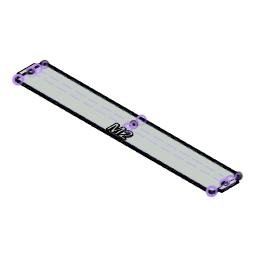
gridfinitybinlabel_parametric_blankPictogram v6 (Autodesk Fusion 360 design; units mm, degrees)
Autodesk Fusion 360 part; units mm, degrees
sketch "Sketch1" plane through (0, 0, 35.65) normal (0, 0, 1) x (-1, 0, 0)
  line L0 (-2.15, 2.65) -> (-39.9, 2.65)
  line L1 (-0.25, -3.35) -> (-0.25, -0.5)
  line L2 (-1.25, -0.5) -> (-1.25, 1.5)
  arc A0 (-1.25, 1.5) -> (-2.15, 2.4) centre (-2.15, 1.5) ccw
  line L3 (-2.15, 2.4) -> (-39.9, 2.4)
  line L4 (-1.25, -0.5) -> (-0.25, -0.5)
  line L5 (0, -3.35) -> (0, 0)
  line L6 (0, 0) -> (-1, 0)
  line L7 (-1, 0) -> (-1, 1.5)
  arc A1 (-1, 1.5) -> (-2.15, 2.65) centre (-2.15, 1.5) ccw
  line L8 (-39.9, -3.35) -> (-39.9, 2.65)
  line L9 (0, -3.35) -> (-39.9, -3.35)
  line L10 (0, 0) -> (-24, 0) construction
  line L11 (0, -3.35) -> (0, -6.7)
  line L12 (-1, -6.7) -> (-1, -8.2)
  line L13 (0, -3.35) -> (-39.9, -3.35)
  line L14 (-1.25, -6.2) -> (-0.25, -6.2)
  arc A2 (-2.15, -9.35) -> (-1, -8.2) centre (-2.15, -8.2) ccw
  line L15 (-2.15, -9.35) -> (-39.9, -9.35)
  line L16 (-1.25, -6.2) -> (-1.25, -8.2)
  line L17 (0, -6.7) -> (-1, -6.7)
  arc A3 (-2.15, -9.1) -> (-1.25, -8.2) centre (-2.15, -8.2) ccw
  line L18 (-0.25, -3.35) -> (-0.25, -6.2)
  line L19 (-2.15, -9.1) -> (-39.9, -9.1)
  line L20 (-39.9, -3.35) -> (-39.9, -9.35)
  line L21 (-78.55, -6.2) -> (-79.55, -6.2)
  line L22 (-79.8, -6.7) -> (-78.8, -6.7)
  line L23 (-77.65, -9.35) -> (-39.9, -9.35)
  line L24 (-79.8, -3.35) -> (-39.9, -3.35)
  line L25 (-78.8, 0) -> (-78.8, 1.5)
  line L26 (-77.65, 2.4) -> (-39.9, 2.4)
  line L27 (-78.55, -0.5) -> (-79.55, -0.5)
  line L28 (-77.65, 2.65) -> (-39.9, 2.65)
  arc A4 (-77.65, 2.4) -> (-78.55, 1.5) centre (-77.65, 1.5) ccw
  line L29 (-79.55, -3.35) -> (-79.55, -6.2)
  line L30 (-79.55, -3.35) -> (-79.55, -0.5)
  line L31 (-79.8, -3.35) -> (-39.9, -3.35)
  line L32 (-78.55, -6.2) -> (-78.55, -8.2)
  arc A5 (-78.55, -8.2) -> (-77.65, -9.1) centre (-77.65, -8.2) ccw
  line L33 (-79.8, -3.35) -> (-79.8, 0)
  line L34 (-39.9, -3.35) -> (-39.9, 2.65)
  line L35 (-79.8, 0) -> (-78.8, 0)
  arc A6 (-77.65, 2.65) -> (-78.8, 1.5) centre (-77.65, 1.5) ccw
  arc A7 (-78.8, -8.2) -> (-77.65, -9.35) centre (-77.65, -8.2) ccw
  line L36 (-78.55, -0.5) -> (-78.55, 1.5)
  line L37 (-77.65, -9.1) -> (-39.9, -9.1)
  line L38 (-78.8, -6.7) -> (-78.8, -8.2)
  line L39 (-39.9, -3.35) -> (-39.9, -9.35)
  line L40 (-79.8, -3.35) -> (-79.8, -6.7)
  point P0 (0, -6.7)
  point P1 (0, -6.7)
  point P2 (-79.8, -6.7)
  point P3 (-79.8, -6.7)
  point P4 (-79.8, 0)
  point P5 (-79.8, 0)
  dimension "d562" = 0.25
  dimension "d566" = 0.5
  dimension "d4" = 39.9
  dimension "d5" = 3.35
  dimension "d6" = 1
  dimension "d7" = 1
  dimension "d8" = 1.15
  dimension "d9" = 0.9
  dimension "d10" = 2
  dimension "d11" = 1.5
  dimension "d12" = 0.9
  dimension "d13" = 1.15
  constraint coincident L1 L4.end
  constraint perpendicular L1 L4
  constraint tangent L2 A0
  constraint tangent A0 L3
  constraint coincident A0.centre A1.centre
  constraint coincident L5.end L6.start
  constraint coincident L8 L3.end
  constraint coincident L9 L1.start
  constraint parallel L0 L3
  constraint perpendicular L6 L7
  constraint perpendicular L5 L9
  constraint parallel L9 L10
  constraint symmetric L5.end L9 P1
  constraint symmetric L0.start L9 A2.start
  constraint symmetric L2.end L9 L16.end
  constraint symmetric A0.end L9 A3.start
  constraint symmetric A0 L9 A3
  constraint symmetric L2.start L9 L14.start
  constraint symmetric L1.end L9 L14.end
  constraint symmetric L6.end L9 L12.start
  constraint symmetric L7.end L9 L12.end
  constraint symmetric A1 L9 A2
  constraint symmetric L5.start L9 L11.start
  constraint symmetric L8.start L9 L13.end
  constraint symmetric L0.end L9 L15.end
  constraint symmetric L3.end L9 L19.end
  constraint symmetric L9 L1.start L18.start
  constraint symmetric L9 L5.end P1
  constraint symmetric L5.end L20 P5
  constraint symmetric L0.start L20 L28.start
  constraint symmetric L2.end L20 A4.end
  constraint symmetric A0.end L20 L26.start
  constraint symmetric A0 L20 A4
  constraint symmetric L2.start L20 L27.start
  constraint symmetric L1.end L20 L27.end
  constraint symmetric L6.end L20 L25.start
  constraint symmetric L7.end L20 L25.end
  constraint symmetric A1 L20 A6
  constraint symmetric L5.start L20 L24.start
  constraint symmetric L8.start L20 L9.end
  constraint symmetric L0.end L20 L8.end
  constraint symmetric L3.end L20 L26.end
  constraint symmetric L1.start L20 L29.start
  constraint symmetric L15.end L20 L23.end
  constraint symmetric A3.start L20 A5.end
  constraint symmetric L12.end L20 A7.start
  constraint symmetric P1 L20 P3
  constraint symmetric L12.start L20 L22.end
  constraint symmetric L19.end L20 L37.end
  constraint symmetric L16.end L20 L32.end
  constraint symmetric L14.end L20 L21.end
  constraint symmetric A2.start L20 L23.start
  constraint symmetric L14.start L20 L21.start
  constraint symmetric A2 L20 A7
  constraint symmetric A3 L20 A5
  constraint perpendicular L3 L34
  measures "d562" distance of L1 L5
  measures "d566" distance of L4 L6
  measures "d4" distance of L5.start L8.start
  measures "d5" distance of L5.end L5.start
  measures "d6" distance of L5.end L6.end
  measures "d7" distance of L2.start L1.end
  measures "d8" radius of A1
  measures "d9" radius of A0
  measures "d10" distance of L2.end L2.start
  measures "d11" distance of L6.end L7.end
  measures "d12" distance of L2 A0.end
  measures "d13" horizontal distance of L0.start L7.end
extrude "Extrude1" add sketch "Sketch1" along normal blind 0.4
sketch "Sketch2" plane through (0, 0, 36.05) normal (0, 0, 1) x (-1, 0, 0)
  line L0 (-2.15, -8.6) -> (-77.65, -8.6)
  line L1 (-78.05, -8.2) -> (-78.05, 1.5)
  line L2 (-77.65, 1.9) -> (-2.15, 1.9)
  line L3 (-1.75, 1.5) -> (-1.75, -8.2)
  arc A0 (-2.15, -8.6) -> (-1.75, -8.2) centre (-2.15, -8.2) ccw
  arc A1 (-1.75, 1.5) -> (-2.15, 1.9) centre (-2.15, 1.5) ccw
  arc A2 (-77.65, 1.9) -> (-78.05, 1.5) centre (-77.65, 1.5) ccw
  arc A3 (-78.05, -8.2) -> (-77.65, -8.6) centre (-77.65, -8.2) ccw
  circle A4 centre (-1.75, -3.35) radius 0.75
  circle A5 centre (-78.05, -3.35) radius 0.75
  circle A6 centre (-1.75, -3.35) radius 1.25
  circle A7 centre (-78.05, -3.35) radius 1.25
  arc A8 (-2.15, -9.35) -> (-1, -8.2) centre (-2.15, -8.2) ccw
  line L4 (-1, -8.2) -> (-1, -6.7)
  line L5 (-1, -6.7) -> (0, -6.7)
  line L6 (0, -6.7) -> (0, 0)
  line L7 (0, 0) -> (-1, 0)
  line L8 (-1, 0) -> (-1, 1.5)
  arc A9 (-1, 1.5) -> (-2.15, 2.65) centre (-2.15, 1.5) ccw
  arc A10 (-77.65, 2.65) -> (-78.8, 1.5) centre (-77.65, 1.5) ccw
  line L9 (-2.15, 2.65) -> (-77.65, 2.65)
  arc A11 (-77.65, 2.65) -> (-78.8, 1.5) centre (-77.65, 1.5) ccw
  line L10 (-78.8, 1.5) -> (-78.8, 0)
  line L11 (-78.8, 0) -> (-79.8, 0)
  line L12 (-79.8, 0) -> (-79.8, -6.7)
  line L13 (-79.8, -6.7) -> (-78.8, -6.7)
  line L14 (-78.8, -6.7) -> (-78.8, -8.2)
  arc A12 (-78.8, -8.2) -> (-77.65, -9.35) centre (-77.65, -8.2) ccw
  line L15 (-77.65, -9.35) -> (-2.15, -9.35)
  point P0 (-2.15, -8.2)
  dimension "d517" = 1.5
  dimension "d518" = 2.5
  constraint horizontal L0
  constraint vertical L1
  constraint horizontal L2
  constraint vertical L3
  constraint tangent L0 A0
  constraint tangent L3 A0
  constraint tangent L3 A1
  constraint tangent L2 A1
  constraint equal A0 A1
  constraint tangent L2 A2
  constraint tangent L1 A2
  constraint equal A0 A2
  constraint tangent L1 A3
  constraint tangent L0 A3
  constraint equal A0 A3
  constraint midpoint L3 A4.centre
  constraint midpoint L1 A5.centre
  constraint concentric A4 A6
  constraint concentric A5 A7
  constraint equal A4 A5
  constraint equal A6 A7
  constraint coincident P0 A0.centre
  constraint concentric A2 A10
  measures "d517" diameter of A4
  measures "d518" diameter of A6
extrude "Extrude2" add sketch "Sketch2" along normal blind 0.4 contours L3 A4 A6 | L3 A4 A6 | L1 A5 A7 | L1 A5 A7 | L3 A4 | L3 A4 | L1 A5 | L1 A5 | A8 L4 L5 L6 L7 L8 A9 A10 L9 A11 L10 L11 L12 L13 L14 A12 L15
fillet "Fillet2" radius 1 6 edges at (1.75, 4.6, 36.25) (1.75, 2.1, 36.25) (1.75, 4.6, 36.25) (1.75, 2.1, 36.25) (78.05, 2.1, 36.25) (78.05, 4.6, 36.25)
extrude "Extrude4" cut sketch "Sketch2" along normal through all and the other way through all contours L3 A4 | L3 A4 | L1 A5 | L1 A5
fillet "Fillet1" radius 0.2 2 faces at (79.4667, 3.35, 36.45) (39.9, 1.35, 35.65)
sketch "Sketch3" plane through (0, 0, 36.05) normal (0, 0, 1) x (-1, 0, 0)
  line L0 (-77.65, -8.6) -> (-2.15, -8.6)
  line L1 (-2.15, 1.9) -> (-77.65, 1.9)
  line L2 (-2.15, -8.6) -> (-77.65, -8.6) construction
  line L3 (-77.65, -8.6) -> (-77.65, 1.9) construction
  line L4 (-77.65, 1.9) -> (-2.15, 1.9) construction
  line L5 (-2.15, 1.9) -> (-2.15, -8.6) construction
  line L6 (-2.15, -3.35) -> (-77.65, -3.35) construction
  arc A0 (-77.4944, -4.4698) -> (-78.05, -5.3656) centre (-77.05, -5.3656) ccw
  line L7 (-78.05, -5.3656) -> (-78.05, -8.2)
  arc A1 (-78.05, -8.2) -> (-77.65, -8.6) centre (-77.65, -8.2) ccw
  arc A2 (-2.15, -8.6) -> (-1.75, -8.2) centre (-2.15, -8.2) ccw
  line L8 (-1.75, -8.2) -> (-1.75, -5.3656)
  arc A3 (-1.75, -5.3656) -> (-2.3056, -4.4698) centre (-2.75, -5.3656) ccw
  arc A4 (-2.3056, -2.2302) -> (-2.3056, -4.4698) centre (-1.75, -3.35) ccw
  arc A5 (-2.3056, -2.2302) -> (-1.75, -1.3344) centre (-2.75, -1.3344) ccw
  line L9 (-1.75, -1.3344) -> (-1.75, 1.5)
  arc A6 (-1.75, 1.5) -> (-2.15, 1.9) centre (-2.15, 1.5) ccw
  arc A7 (-77.65, 1.9) -> (-78.05, 1.5) centre (-77.65, 1.5) ccw
  line L10 (-78.05, 1.5) -> (-78.05, -1.3344)
  arc A8 (-78.05, -1.3344) -> (-77.4944, -2.2302) centre (-77.05, -1.3344) ccw
  arc A9 (-77.4944, -4.4698) -> (-77.4944, -2.2302) centre (-78.05, -3.35) ccw
  line L11 (-2.15, -5.6) -> (-77.65, -5.6) construction
  line L12 (-39.9, -8.6) -> (-39.9, -5.6) construction
  line L13 (-39.9, -5.6) -> (-39.9, -3.35) construction
  line L14 (-34.3, -5.6) -> (-13, -5.6)
  line L15 (-13, -5.6) -> (-10, -5.6)
  line L16 (-2.15, 1.5) -> (-77.65, 1.5) construction
  line L17 (-77.65, 1.5) -> (-77.65, -3.35) construction
  line L18 (-77.65, -3.35) -> (-2.15, -3.35) construction
  line L19 (-2.15, -3.35) -> (-2.15, 1.5) construction
  line L20 (-39.9, -2.6) -> (-39.9, -5.6) construction
  line L21 (-13, -5.6) -> (-10, -5.6)
  point P0 (-34.3, -6.85)
  point P1 (-10, -8.1)
  point P2 (-6, -5.6)
  point P3 (-10, -3.1)
  point P4 (-34.3, -4.35)
  dimension "d21" = 3
  dimension "d22" = 0.4
  dimension "d26" = 2.5
  dimension "d38" = 75.5
  dimension "d43" = 4
  dimension "d44" = 0.4
  dimension "d67" = 0.4
  constraint horizontal L2
  constraint vertical L3
  constraint horizontal L4
  constraint vertical L5
  constraint midpoint L5 L6.start
  constraint midpoint L3 L6.end
  constraint coincident L5 L11.start
  constraint coincident L3 L11.end
  constraint perpendicular L3 L11
  constraint midpoint L2 L12.start
  constraint midpoint L11 L12.end
  constraint horizontal L14
  constraint coincident L11 L14.start
  constraint horizontal L15
  constraint coincident L1.start L4
  constraint coincident L5
  constraint coincident L6.end
  constraint symmetric L11 L12.start L20.start
  constraint symmetric L11 L12.end L13.start
  constraint symmetric L11 L14.end L15.start
  constraint symmetric L11 P0 P4
  constraint symmetric L11 L15.end L21.end
  constraint symmetric L11 P1 P3
  measures "d21" distance of L0 L11
  measures "d22" distance of L8 L11.start
  measures "d26" distance of L15.end P1
  measures "d38" distance of L0.end L0.start
  measures "d44" distance of L4 L16
  measures "d67" distance of L3 L7
sketch "Main Construction Geometry" plane through (0, 0, 36.05) normal (0, 0, 1) x (-1, 0, 0)
  arc A0 (-77.4944, -4.4698) -> (-78.05, -5.3656) centre (-77.05, -5.3656) ccw construction
  line L0 (-78.05, -5.3656) -> (-78.05, -8.2) construction
  arc A1 (-78.05, -8.2) -> (-77.65, -8.6) centre (-77.65, -8.2) ccw construction
  line L1 (-77.65, -8.6) -> (-2.15, -8.6) construction
  arc A2 (-2.15, -8.6) -> (-1.75, -8.2) centre (-2.15, -8.2) ccw construction
  line L2 (-1.75, -8.2) -> (-1.75, -5.3656) construction
  arc A3 (-1.75, -5.3656) -> (-2.3056, -4.4698) centre (-2.75, -5.3656) ccw construction
  arc A4 (-2.3056, -2.2302) -> (-2.3056, -4.4698) centre (-1.75, -3.35) ccw construction
  arc A5 (-2.3056, -2.2302) -> (-1.75, -1.3344) centre (-2.75, -1.3344) ccw construction
  line L3 (-1.75, -1.3344) -> (-1.75, 1.5) construction
  arc A6 (-1.75, 1.5) -> (-2.15, 1.9) centre (-2.15, 1.5) ccw construction
  line L4 (-2.15, 1.9) -> (-77.65, 1.9) construction
  arc A7 (-77.65, 1.9) -> (-78.05, 1.5) centre (-77.65, 1.5) ccw construction
  line L5 (-78.05, 1.5) -> (-78.05, -1.3344) construction
  arc A8 (-78.05, -1.3344) -> (-77.4944, -2.2302) centre (-77.05, -1.3344) ccw construction
  arc A9 (-77.4944, -4.4698) -> (-77.4944, -2.2302) centre (-78.05, -3.35) ccw construction
  line L6 (-2.15, -5.6) -> (-77.65, -5.6) construction
  line L7 (-2.15, 1.9) -> (-2.15, -8.6) construction
  line L8 (-2.15, -8.6) -> (-77.65, -8.6) construction
  line L9 (-39.9, -8.6) -> (-39.9, -5.6) construction
  line L10 (-39.9, -5.6) -> (-39.9, -3.35) construction
  line L11 (-2.15, -3.35) -> (-77.65, -3.35) construction
  line L12 (-77.65, -8.6) -> (-77.65, 1.9) construction
  line L13 (-2.15, 1.5) -> (-77.65, 1.5) construction
sketch "Pictogram" plane through (0, 0, 36.05) normal (0, 0, 1) x (-1, 0, 0)
  arc A0 (-77.4944, -4.4698) -> (-78.05, -5.3656) centre (-77.05, -5.3656) ccw
  line L0 (-78.05, -5.3656) -> (-78.05, -8.2)
  arc A1 (-78.05, -8.2) -> (-77.65, -8.6) centre (-77.65, -8.2) ccw
  line L1 (-77.65, -8.6) -> (-2.15, -8.6)
  arc A2 (-2.15, -8.6) -> (-1.75, -8.2) centre (-2.15, -8.2) ccw
  line L2 (-1.75, -8.2) -> (-1.75, -5.3656)
  arc A3 (-1.75, -5.3656) -> (-2.3056, -4.4698) centre (-2.75, -5.3656) ccw
  arc A4 (-2.3056, -2.2302) -> (-2.3056, -4.4698) centre (-1.75, -3.35) ccw
  arc A5 (-2.3056, -2.2302) -> (-1.75, -1.3344) centre (-2.75, -1.3344) ccw
  line L3 (-1.75, -1.3344) -> (-1.75, 1.5)
  arc A6 (-1.75, 1.5) -> (-2.15, 1.9) centre (-2.15, 1.5) ccw
  line L4 (-2.15, 1.9) -> (-77.65, 1.9)
  arc A7 (-77.65, 1.9) -> (-78.05, 1.5) centre (-77.65, 1.5) ccw
  line L5 (-78.05, 1.5) -> (-78.05, -1.3344)
  arc A8 (-78.05, -1.3344) -> (-77.4944, -2.2302) centre (-77.05, -1.3344) ccw
  arc A9 (-77.4944, -4.4698) -> (-77.4944, -2.2302) centre (-78.05, -3.35) ccw
sketch "Text" plane through (0, 0, 36.05) normal (0, 0, 1) x (-1, 0, 0)
  arc A0 (-77.4944, -4.4698) -> (-78.05, -5.3656) centre (-77.05, -5.3656) ccw
  line L0 (-78.05, -5.3656) -> (-78.05, -8.2)
  arc A1 (-78.05, -8.2) -> (-77.65, -8.6) centre (-77.65, -8.2) ccw
  line L1 (-77.65, -8.6) -> (-2.15, -8.6)
  arc A2 (-2.15, -8.6) -> (-1.75, -8.2) centre (-2.15, -8.2) ccw
  line L2 (-1.75, -8.2) -> (-1.75, -5.3656)
  arc A3 (-1.75, -5.3656) -> (-2.3056, -4.4698) centre (-2.75, -5.3656) ccw
  arc A4 (-2.3056, -2.2302) -> (-2.3056, -4.4698) centre (-1.75, -3.35) ccw
  arc A5 (-2.3056, -2.2302) -> (-1.75, -1.3344) centre (-2.75, -1.3344) ccw
  line L3 (-1.75, -1.3344) -> (-1.75, 1.5)
  arc A6 (-1.75, 1.5) -> (-2.15, 1.9) centre (-2.15, 1.5) ccw
  line L4 (-2.15, 1.9) -> (-77.65, 1.9)
  arc A7 (-77.65, 1.9) -> (-78.05, 1.5) centre (-77.65, 1.5) ccw
  line L5 (-78.05, 1.5) -> (-78.05, -1.3344)
  arc A8 (-78.05, -1.3344) -> (-77.4944, -2.2302) centre (-77.05, -1.3344) ccw
  arc A9 (-77.4944, -4.4698) -> (-77.4944, -2.2302) centre (-78.05, -3.35) ccw
  line L6 (-2.15, 1.5) -> (-77.65, 1.5) construction
  line L7 (-77.65, 1.5) -> (-77.65, -2.2355) construction
  line L8 (-77.65, -2.2355) -> (-2.15, -2.2355) construction
  line L9 (-2.15, -2.2355) -> (-2.15, 1.5) construction
  point P0 (-2.15, 1.5)
  point P1 (-77.65, 1.5)
  dimension "text_height" = 4
  text T0 "M2" font "Arial" height 4 bold align centre middle in box 75.5 x 3.7355 at (-2.15, 1.5) x (-1, 0) y (0, -1) spacing 1 kerned
  constraint coincident P0
  constraint coincident P1
extrude "Extrude6" add sketch "Text" along normal up to surface (0.4 mm away) text T0
extrude "Extrude3" [suppressed]
sketch "Skizze4" plane through (0, 0, 36.45) normal (0, 0, 1) x (-1, 0, 0)
  line L0 (-12.988, -6.85) -> (-12.988, -5.6) construction
  line L1 (-12.988, -5.6) -> (-34.3, -5.6) construction
  spline S0 degree 5 poles (-23.398, -6.85) (-23.3526, -6.8257) (-23.2673, -6.7758) (-23.156, -6.6971) (-23.0412, -6.5844) (-22.9541, -6.4303) (-22.9227, -6.2632) (-22.9431, -6.0841) (-23.0069, -5.8949) (-23.099, -5.6991) (-23.201, -5.5009) (-23.2931, -5.3051) (-23.3569, -5.1159) (-23.3773, -4.9368) (-23.3459, -4.7697) (-23.2588, -4.6156) (-23.144, -4.5029) (-23.0327, -4.4242) (-22.9474, -4.3743) (-22.902, -4.35) knots 0 0 0 0 0 0 0.066667 0.133333 0.2 0.266667 0.333333 0.4 0.466667 0.533333 0.6 0.666667 0.733333 0.8 0.866667 0.933333 1 1 1 1 1 1
  spline S1 degree 5 poles (-24.398, -6.85) (-24.3526, -6.8257) (-24.2673, -6.7758) (-24.156, -6.6971) (-24.0412, -6.5844) (-23.9541, -6.4303) (-23.9227, -6.2632) (-23.9431, -6.0841) (-24.0069, -5.8949) (-24.099, -5.6991) (-24.201, -5.5009) (-24.2931, -5.3051) (-24.3569, -5.1159) (-24.3773, -4.9368) (-24.3459, -4.7697) (-24.2588, -4.6156) (-24.144, -4.5029) (-24.0327, -4.4242) (-23.9474, -4.3743) (-23.902, -4.35) knots 0 0 0 0 0 0 0.066667 0.133333 0.2 0.266667 0.333333 0.4 0.466667 0.533333 0.6 0.666667 0.733333 0.8 0.866667 0.933333 1 1 1 1 1 1
  line L2 (-23.65, -5.6) -> (-22.95, -6.1)
  line L3 (-23.65, -5.6) -> (-23.95, -6.1)
  line L4 (-24.35, -5.1) -> (-23.65, -5.6)
  line L5 (-23.35, -5.1) -> (-23.65, -5.6)
  line L6 (-12.988, -5.6) -> (-12.988, -4.35) construction
  line L7 (-23.398, -6.85) -> (-24.398, -6.85)
  line L8 (-22.902, -4.35) -> (-23.902, -4.35)
  spline S2 degree 3 poles (-14.6415, -0.0138) (-14.6392, -0.1132) (-14.6345, -0.3083) (-14.5979, -0.4999) (-14.58, -0.5938) knots -0.058414 -0.058414 -0.058414 -0.058414 -0.028644 0 0 0 0
  spline S3 degree 3 poles (-14.58, -0.5938) (-14.5573, -0.6814) (-14.5135, -0.8507) (-14.4265, -1.0023) (-14.3846, -1.0754) knots -0.052175 -0.052175 -0.052175 -0.052175 -0.025167 0 0 0 0
  spline S4 degree 3 poles (-14.3846, -1.0754) (-14.3368, -1.1406) (-14.2412, -1.2707) (-14.106, -1.359) (-14.0385, -1.4031) knots -0.048014 -0.048014 -0.048014 -0.048014 -0.023977 0 0 0 0
  spline S5 degree 3 poles (-14.0385, -1.4031) (-13.9612, -1.4385) (-13.7973, -1.5136) (-13.6169, -1.5208) (-13.5215, -1.5246) knots -0.053559 -0.053559 -0.053559 -0.053559 -0.028317 0 0 0 0
  spline S6 degree 3 poles (-13.5215, -1.5246) (-13.4814, -1.5238) (-13.403, -1.5222) (-13.3256, -1.5094) (-13.2877, -1.5031) knots -0.023511 -0.023511 -0.023511 -0.023511 -0.011499 0 0 0 0
  spline S7 degree 3 poles (-13.2877, -1.5031) (-13.2509, -1.4948) (-13.1771, -1.4781) (-13.1073, -1.4486) (-13.0723, -1.4338) knots -0.022663 -0.022663 -0.022663 -0.022663 -0.011385 0 0 0 0
  spline S8 degree 3 poles (-13.0723, -1.4338) (-13.037, -1.4165) (-12.9644, -1.381) (-12.8975, -1.3356) (-12.8631, -1.3123) knots -0.024223 -0.024223 -0.024223 -0.024223 -0.01244 0 0 0 0
  spline S9 degree 3 poles (-12.8631, -1.3123) (-12.8276, -1.2858) (-12.754, -1.2309) (-12.688, -1.167) (-12.6538, -1.1338) knots -0.027525 -0.027525 -0.027525 -0.027525 -0.014261 0 0 0 0
  line L9 (-12.6538, -1.1338) -> (-12.6538, -2.6508)
  spline S10 degree 3 poles (-12.6538, -2.6508) (-12.6531, -2.6608) (-12.6515, -2.6808) (-12.6408, -2.6977) (-12.6354, -2.7062) knots -0.005919 -0.005919 -0.005919 -0.005919 -0.002959 0 0 0 0
  spline S11 degree 3 poles (-12.6354, -2.7062) (-12.6274, -2.7143) (-12.6095, -2.7327) (-12.5856, -2.7423) (-12.5723, -2.7477) knots -0.007625 -0.007625 -0.007625 -0.007625 -0.004249 0 0 0 0
  spline S12 degree 3 poles (-12.5723, -2.7477) (-12.5551, -2.7531) (-12.5164, -2.7654) (-12.4762, -2.7708) (-12.4538, -2.7738) knots -0.012151 -0.012151 -0.012151 -0.012151 -0.006747 0 0 0 0
  spline S13 degree 3 poles (-12.4538, -2.7738) (-12.4259, -2.7765) (-12.3635, -2.7825) (-12.3008, -2.7829) (-12.2662, -2.7831) knots -0.0188 -0.0188 -0.0188 -0.0188 -0.010387 0 0 0 0
  spline S14 degree 3 poles (-12.2662, -2.7831) (-12.2315, -2.7829) (-12.1688, -2.7825) (-12.1064, -2.7765) (-12.0785, -2.7738) knots -0.0188 -0.0188 -0.0188 -0.0188 -0.008413 0 0 0 0
  spline S15 degree 3 poles (-12.0785, -2.7738) (-12.0561, -2.7708) (-12.0159, -2.7654) (-11.9772, -2.7531) (-11.96, -2.7477) knots -0.012151 -0.012151 -0.012151 -0.012151 -0.005405 0 0 0 0
  spline S16 degree 3 poles (-11.96, -2.7477) (-11.9467, -2.7423) (-11.9228, -2.7327) (-11.9049, -2.7143) (-11.8969, -2.7062) knots -0.007625 -0.007625 -0.007625 -0.007625 -0.003376 0 0 0 0
  spline S17 degree 3 poles (-11.8969, -2.7062) (-11.8915, -2.6977) (-11.8808, -2.6808) (-11.8792, -2.6608) (-11.8785, -2.6508) knots -0.005919 -0.005919 -0.005919 -0.005919 -0.002959 0 0 0 0
  line L10 (-11.8785, -2.6508) -> (-11.8785, 1.3954)
  spline S18 degree 3 poles (-11.8785, 1.3954) (-11.879, 1.406) (-11.8799, 1.4261) (-11.8894, 1.4439) (-11.8938, 1.4523) knots -0.005963 -0.005963 -0.005963 -0.005963 -0.002824 0 0 0 0
  spline S19 degree 3 poles (-11.8938, 1.4523) (-11.9005, 1.4599) (-11.9154, 1.4769) (-11.9362, 1.4858) (-11.9477, 1.4908) knots -0.006691 -0.006691 -0.006691 -0.006691 -0.003699 0 0 0 0
  spline S20 degree 3 poles (-11.9477, 1.4908) (-11.9625, 1.4956) (-11.9955, 1.5064) (-12.0301, 1.5102) (-12.0492, 1.5123) knots -0.010404 -0.010404 -0.010404 -0.010404 -0.005755 0 0 0 0
  spline S21 degree 3 poles (-12.0492, 1.5123) (-12.0729, 1.5141) (-12.1257, 1.5181) (-12.1786, 1.5183) (-12.2077, 1.5185) knots -0.015862 -0.015862 -0.015862 -0.015862 -0.008732 0 0 0 0
  spline S22 degree 3 poles (-12.2077, 1.5185) (-12.2362, 1.5183) (-12.2885, 1.518) (-12.3408, 1.5141) (-12.3646, 1.5123) knots -0.015709 -0.015709 -0.015709 -0.015709 -0.007169 0 0 0 0
  spline S23 degree 3 poles (-12.3646, 1.5123) (-12.3841, 1.5102) (-12.4192, 1.5065) (-12.4528, 1.4956) (-12.4677, 1.4908) knots -0.010555 -0.010555 -0.010555 -0.010555 -0.004686 0 0 0 0
  spline S24 degree 3 poles (-12.4677, 1.4908) (-12.4793, 1.4858) (-12.5004, 1.4766) (-12.516, 1.4599) (-12.5231, 1.4523) knots -0.006807 -0.006807 -0.006807 -0.006807 -0.003074 0 0 0 0
  spline S25 degree 3 poles (-12.5231, 1.4523) (-12.528, 1.4439) (-12.5383, 1.4264) (-12.5394, 1.406) (-12.54, 1.3954) knots -0.006017 -0.006017 -0.006017 -0.006017 -0.003144 0 0 0 0
  line L11 (-12.54, 1.3954) -> (-12.54, 1.0969)
  spline S26 degree 3 poles (-12.54, 1.0969) (-12.5758, 1.1366) (-12.6441, 1.2125) (-12.7205, 1.2801) (-12.7569, 1.3123) knots -0.030591 -0.030591 -0.030591 -0.030591 -0.014564 0 0 0 0
  spline S27 degree 3 poles (-12.7569, 1.3123) (-12.7919, 1.3405) (-12.8599, 1.3953) (-12.9356, 1.4388) (-12.9723, 1.46) knots -0.026151 -0.026151 -0.026151 -0.026151 -0.012704 0 0 0 0
  spline S28 degree 3 poles (-12.9723, 1.46) (-13.0091, 1.4781) (-13.0826, 1.5143) (-13.1619, 1.5345) (-13.2015, 1.5446) knots -0.024494 -0.024494 -0.024494 -0.024494 -0.01222 0 0 0 0
  spline S29 degree 3 poles (-13.2015, 1.5446) (-13.243, 1.5522) (-13.3284, 1.568) (-13.4153, 1.5698) (-13.46, 1.5708) knots -0.026016 -0.026016 -0.026016 -0.026016 -0.013401 0 0 0 0
  spline S30 degree 3 poles (-13.46, 1.5708) (-13.5495, 1.5668) (-13.7228, 1.5591) (-13.8827, 1.4923) (-13.96, 1.46) knots -0.05157 -0.05157 -0.05157 -0.05157 -0.024925 0 0 0 0
  spline S31 degree 3 poles (-13.96, 1.46) (-14.0307, 1.4188) (-14.1734, 1.3356) (-14.278, 1.2076) (-14.3308, 1.1431) knots -0.049129 -0.049129 -0.049129 -0.049129 -0.024796 0 0 0 0
  spline S32 degree 3 poles (-14.3308, 1.1431) (-14.3786, 1.0688) (-14.4786, 0.9135) (-14.5331, 0.7368) (-14.5615, 0.6446) knots -0.055158 -0.055158 -0.055158 -0.055158 -0.028785 0 0 0 0
  spline S33 degree 3 poles (-14.5615, 0.6446) (-14.5849, 0.5414) (-14.6338, 0.3247) (-14.6389, 0.1026) (-14.6415, -0.0138) knots -0.066478 -0.066478 -0.066478 -0.066478 -0.034827 0 0 0 0
  spline S34 degree 3 poles (-13.8385, 0.0415) (-13.8372, 0.094) (-13.8345, 0.1993) (-13.8167, 0.3032) (-13.8077, 0.3554) knots -0.031572 -0.031572 -0.031572 -0.031572 -0.015861 0 0 0 0
  spline S35 degree 3 poles (-13.8077, 0.3554) (-13.7962, 0.4056) (-13.774, 0.5029) (-13.7293, 0.5922) (-13.7077, 0.6354) knots -0.029827 -0.029827 -0.029827 -0.029827 -0.014442 0 0 0 0
  spline S36 degree 3 poles (-13.7077, 0.6354) (-13.6835, 0.6742) (-13.6362, 0.7502) (-13.5675, 0.8074) (-13.5338, 0.8354) knots -0.026652 -0.026652 -0.026652 -0.026652 -0.013037 0 0 0 0
  spline S37 degree 3 poles (-13.5338, 0.8354) (-13.4961, 0.8578) (-13.4175, 0.9045) (-13.326, 0.9096) (-13.2785, 0.9123) knots -0.027024 -0.027024 -0.027024 -0.027024 -0.014055 0 0 0 0
  spline S38 degree 3 poles (-13.2785, 0.9123) (-13.2239, 0.9072) (-13.1109, 0.8965) (-13.0155, 0.8349) (-12.9662, 0.8031) knots -0.033522 -0.033522 -0.033522 -0.033522 -0.017328 0 0 0 0
  spline S39 degree 3 poles (-12.9662, 0.8031) (-12.9138, 0.7598) (-12.7986, 0.6647) (-12.7049, 0.5481) (-12.6538, 0.4846) knots -0.044706 -0.044706 -0.044706 -0.044706 -0.024376 0 0 0 0
  line L12 (-12.6538, 0.4846) -> (-12.6538, -0.4262)
  spline S40 degree 3 poles (-12.6538, -0.4262) (-12.6832, -0.4644) (-12.7381, -0.5362) (-12.8002, -0.6017) (-12.8292, -0.6323) knots -0.027083 -0.027083 -0.027083 -0.027083 -0.012631 0 0 0 0
  spline S41 degree 3 poles (-12.8292, -0.6323) (-12.8559, -0.6582) (-12.9065, -0.7072) (-12.9637, -0.7483) (-12.9908, -0.7677) knots -0.021102 -0.021102 -0.021102 -0.021102 -0.009969 0 0 0 0
  spline S42 degree 3 poles (-12.9908, -0.7677) (-13.016, -0.7836) (-13.0641, -0.814) (-13.1177, -0.8327) (-13.1431, -0.8415) knots -0.016975 -0.016975 -0.016975 -0.016975 -0.00805 0 0 0 0
  spline S43 degree 3 poles (-13.1431, -0.8415) (-13.1678, -0.8478) (-13.2173, -0.8604) (-13.2683, -0.8622) (-13.2938, -0.8631) knots -0.015269 -0.015269 -0.015269 -0.015269 -0.007634 0 0 0 0
  spline S44 degree 3 poles (-13.2938, -0.8631) (-13.3428, -0.8607) (-13.4357, -0.8562) (-13.5159, -0.8097) (-13.5538, -0.7877) knots -0.027422 -0.027422 -0.027422 -0.027422 -0.012953 0 0 0 0
  spline S45 degree 3 poles (-13.5538, -0.7877) (-13.5869, -0.7599) (-13.6548, -0.7028) (-13.6989, -0.6257) (-13.7215, -0.5862) knots -0.026401 -0.026401 -0.026401 -0.026401 -0.013559 0 0 0 0
  spline S46 degree 3 poles (-13.7215, -0.5862) (-13.7416, -0.5416) (-13.7834, -0.4488) (-13.8024, -0.3489) (-13.8123, -0.2969) knots -0.030408 -0.030408 -0.030408 -0.030408 -0.015795 0 0 0 0
  spline S47 degree 3 poles (-13.8123, -0.2969) (-13.8199, -0.2416) (-13.8354, -0.1293) (-13.8374, -0.016) (-13.8385, 0.0415) knots -0.033974 -0.033974 -0.033974 -0.033974 -0.017243 0 0 0 0
  line L13 (-19.1462, 1.4046) -> (-19.1462, -0.4415)
  spline S48 degree 3 poles (-19.1462, -0.4415) (-19.1442, -0.53) (-19.1405, -0.6958) (-19.0982, -0.856) (-19.0785, -0.9308) knots -0.049542 -0.049542 -0.049542 -0.049542 -0.023103 0 0 0 0
  spline S49 degree 3 poles (-19.0785, -0.9308) (-19.0532, -0.9958) (-19.0039, -1.1226) (-18.9092, -1.2201) (-18.8631, -1.2677) knots -0.040352 -0.040352 -0.040352 -0.040352 -0.01967 0 0 0 0
  spline S50 degree 3 poles (-18.8631, -1.2677) (-18.8088, -1.3089) (-18.6946, -1.3955) (-18.5578, -1.4388) (-18.4862, -1.4615) knots -0.042665 -0.042665 -0.042665 -0.042665 -0.022364 0 0 0 0
  spline S51 degree 3 poles (-18.4862, -1.4615) (-18.4022, -1.4799) (-18.2204, -1.5197) (-18.0341, -1.5229) (-17.9338, -1.5246) knots -0.055711 -0.055711 -0.055711 -0.055711 -0.030003 0 0 0 0
  spline S52 degree 3 poles (-17.9338, -1.5246) (-17.8741, -1.5235) (-17.7561, -1.5212) (-17.6393, -1.5039) (-17.5815, -1.4954) knots -0.035384 -0.035384 -0.035384 -0.035384 -0.017484 0 0 0 0
  spline S53 degree 3 poles (-17.5815, -1.4954) (-17.5266, -1.4852) (-17.4201, -1.4655) (-17.3163, -1.4348) (-17.2662, -1.42) knots -0.032447 -0.032447 -0.032447 -0.032447 -0.015686 0 0 0 0
  spline S54 degree 3 poles (-17.2662, -1.42) (-17.2207, -1.4049) (-17.1347, -1.3763) (-17.0525, -1.338) (-17.0138, -1.32) knots -0.02716 -0.02716 -0.02716 -0.02716 -0.012793 0 0 0 0
  spline S55 degree 3 poles (-17.0138, -1.32) (-16.9824, -1.3041) (-16.9284, -1.2769) (-16.8824, -1.2379) (-16.8631, -1.2215) knots -0.018062 -0.018062 -0.018062 -0.018062 -0.007557 0 0 0 0
  spline S56 degree 3 poles (-16.8631, -1.2215) (-16.8499, -1.2064) (-16.8241, -1.1767) (-16.811, -1.1397) (-16.8046, -1.1215) knots -0.011676 -0.011676 -0.011676 -0.011676 -0.005722 0 0 0 0
  spline S57 degree 3 poles (-16.8046, -1.1215) (-16.8001, -1.0998) (-16.7899, -1.0501) (-16.7895, -0.9993) (-16.7892, -0.9708) knots -0.015187 -0.015187 -0.015187 -0.015187 -0.008547 0 0 0 0
  spline S58 degree 3 poles (-16.7892, -0.9708) (-16.7895, -0.9482) (-16.7901, -0.9049) (-16.7958, -0.862) (-16.7985, -0.8415) knots -0.012966 -0.012966 -0.012966 -0.012966 -0.006193 0 0 0 0
  spline S59 degree 3 poles (-16.7985, -0.8415) (-16.8016, -0.8234) (-16.8074, -0.7898) (-16.8192, -0.7578) (-16.8246, -0.7431) knots -0.010206 -0.010206 -0.010206 -0.010206 -0.004707 0 0 0 0
  spline S60 degree 3 poles (-16.8246, -0.7431) (-16.8303, -0.7308) (-16.8411, -0.7077) (-16.8592, -0.6899) (-16.8677, -0.6815) knots -0.007567 -0.007567 -0.007567 -0.007567 -0.003539 0 0 0 0
  spline S61 degree 3 poles (-16.8677, -0.6815) (-16.8767, -0.6753) (-16.8948, -0.6627) (-16.9167, -0.6609) (-16.9277, -0.66) knots -0.006477 -0.006477 -0.006477 -0.006477 -0.003238 0 0 0 0
  spline S62 degree 3 poles (-16.9277, -0.66) (-16.9468, -0.6627) (-16.992, -0.669) (-17.0322, -0.6906) (-17.0554, -0.7031) knots -0.01357 -0.01357 -0.01357 -0.01357 -0.007814 0 0 0 0
  spline S63 degree 3 poles (-17.0554, -0.7031) (-17.0846, -0.7185) (-17.1488, -0.7523) (-17.2148, -0.7822) (-17.2508, -0.7985) knots -0.021747 -0.021747 -0.021747 -0.021747 -0.011839 0 0 0 0
  spline S64 degree 3 poles (-17.2508, -0.7985) (-17.2924, -0.8159) (-17.3804, -0.8526) (-17.4719, -0.8796) (-17.52, -0.8938) knots -0.028581 -0.028581 -0.028581 -0.028581 -0.015047 0 0 0 0
  spline S65 degree 3 poles (-17.52, -0.8938) (-17.574, -0.9064) (-17.6878, -0.9329) (-17.8047, -0.9355) (-17.8662, -0.9369) knots -0.034965 -0.034965 -0.034965 -0.034965 -0.018378 0 0 0 0
  spline S66 degree 3 poles (-17.8662, -0.9369) (-17.9116, -0.9361) (-17.9954, -0.9347) (-18.0767, -0.9151) (-18.1138, -0.9062) knots -0.025026 -0.025026 -0.025026 -0.025026 -0.011428 0 0 0 0
  spline S67 degree 3 poles (-18.1138, -0.9062) (-18.145, -0.895) (-18.2047, -0.8737) (-18.2515, -0.8311) (-18.2738, -0.8108) knots -0.018792 -0.018792 -0.018792 -0.018792 -0.008974 0 0 0 0
  spline S68 degree 3 poles (-18.2738, -0.8108) (-18.2926, -0.7874) (-18.3313, -0.7389) (-18.3502, -0.6798) (-18.36, -0.6492) knots -0.018446 -0.018446 -0.018446 -0.018446 -0.009535 0 0 0 0
  spline S69 degree 3 poles (-18.36, -0.6492) (-18.3676, -0.6144) (-18.3839, -0.5399) (-18.3854, -0.4636) (-18.3862, -0.4231) knots -0.022815 -0.022815 -0.022815 -0.022815 -0.012133 0 0 0 0
  line L14 (-18.3862, -0.4231) -> (-18.3862, -0.2569)
  line L15 (-18.3862, -0.2569) -> (-18.1185, -0.2569)
  spline S70 degree 3 poles (-18.1185, -0.2569) (-18.0036, -0.2553) (-17.7878, -0.2522) (-17.5749, -0.2177) (-17.4754, -0.2015) knots -0.064622 -0.064622 -0.064622 -0.064622 -0.03021 0 0 0 0
  spline S71 degree 3 poles (-17.4754, -0.2015) (-17.3892, -0.182) (-17.2272, -0.1452) (-17.0808, -0.0672) (-17.0123, -0.0308) knots -0.049551 -0.049551 -0.049551 -0.049551 -0.023172 0 0 0 0
  spline S72 degree 3 poles (-17.0123, -0.0308) (-16.9545, 0.0095) (-16.8415, 0.0883) (-16.7681, 0.2047) (-16.7323, 0.2615) knots -0.040845 -0.040845 -0.040845 -0.040845 -0.019941 0 0 0 0
  spline S73 degree 3 poles (-16.7323, 0.2615) (-16.705, 0.3249) (-16.6475, 0.4578) (-16.6416, 0.6026) (-16.6385, 0.6785) knots -0.04306 -0.04306 -0.04306 -0.04306 -0.022545 0 0 0 0
  spline S74 degree 3 poles (-16.6385, 0.6785) (-16.6409, 0.7484) (-16.6454, 0.8816) (-16.6908, 1.0068) (-16.7123, 1.0662) knots -0.039684 -0.039684 -0.039684 -0.039684 -0.018833 0 0 0 0
  spline S75 degree 3 poles (-16.7123, 1.0662) (-16.7392, 1.1191) (-16.7924, 1.2239) (-16.8778, 1.3047) (-16.92, 1.3446) knots -0.03497 -0.03497 -0.03497 -0.03497 -0.017304 0 0 0 0
  spline S76 degree 3 poles (-16.92, 1.3446) (-16.9674, 1.38) (-17.0644, 1.4524) (-17.1785, 1.493) (-17.2369, 1.5138) knots -0.036108 -0.036108 -0.036108 -0.036108 -0.018485 0 0 0 0
  spline S77 degree 3 poles (-17.2369, 1.5138) (-17.3006, 1.5304) (-17.4322, 1.5648) (-17.5682, 1.5687) (-17.6385, 1.5708) knots -0.040671 -0.040671 -0.040671 -0.040671 -0.02101 0 0 0 0
  spline S78 degree 3 poles (-17.6385, 1.5708) (-17.7237, 1.567) (-17.8899, 1.5596) (-18.0446, 1.4988) (-18.12, 1.4692) knots -0.049515 -0.049515 -0.049515 -0.049515 -0.024118 0 0 0 0
  spline S79 degree 3 poles (-18.12, 1.4692) (-18.1906, 1.4318) (-18.333, 1.3562) (-18.4481, 1.2432) (-18.5062, 1.1862) knots -0.048104 -0.048104 -0.048104 -0.048104 -0.024272 0 0 0 0
  line L16 (-18.5062, 1.1862) -> (-18.5062, 1.4046)
  spline S80 degree 3 poles (-18.5062, 1.4046) (-18.507, 1.418) (-18.5086, 1.4434) (-18.5247, 1.463) (-18.5323, 1.4723) knots -0.007422 -0.007422 -0.007422 -0.007422 -0.00352 0 0 0 0
  spline S81 degree 3 poles (-18.5323, 1.4723) (-18.5438, 1.4801) (-18.5708, 1.4985) (-18.603, 1.5043) (-18.6215, 1.5077) knots -0.009692 -0.009692 -0.009692 -0.009692 -0.00557 0 0 0 0
  spline S82 degree 3 poles (-18.6215, 1.5077) (-18.6488, 1.5108) (-18.7158, 1.5184) (-18.7832, 1.5185) (-18.8231, 1.5185) knots -0.020197 -0.020197 -0.020197 -0.020197 -0.011965 0 0 0 0
  spline S83 degree 3 poles (-18.8231, 1.5185) (-18.8609, 1.5184) (-18.9263, 1.5182) (-18.9912, 1.5108) (-19.0185, 1.5077) knots -0.019581 -0.019581 -0.019581 -0.019581 -0.008232 0 0 0 0
  spline S84 degree 3 poles (-19.0185, 1.5077) (-19.0381, 1.5042) (-19.0726, 1.4981) (-19.1025, 1.4801) (-19.1154, 1.4723) knots -0.010396 -0.010396 -0.010396 -0.010396 -0.004491 0 0 0 0
  spline S85 degree 3 poles (-19.1154, 1.4723) (-19.1244, 1.4632) (-19.1428, 1.4444) (-19.145, 1.4181) (-19.1462, 1.4046) knots -0.007647 -0.007647 -0.007647 -0.007647 -0.003922 0 0 0 0
  line L17 (-18.3862, 0.2292) -> (-18.3862, 0.6969)
  spline S86 degree 3 poles (-18.3862, 0.6969) (-18.3411, 0.7458) (-18.2571, 0.8371) (-18.155, 0.9074) (-18.1077, 0.94) knots -0.037065 -0.037065 -0.037065 -0.037065 -0.017185 0 0 0 0
  spline S87 degree 3 poles (-18.1077, 0.94) (-18.0608, 0.9642) (-17.9667, 1.0129) (-17.8609, 1.0197) (-17.8077, 1.0231) knots -0.031432 -0.031432 -0.031432 -0.031432 -0.015791 0 0 0 0
  spline S88 degree 3 poles (-17.8077, 1.0231) (-17.7483, 1.0204) (-17.6378, 1.0153) (-17.5467, 0.9533) (-17.5046, 0.9246) knots -0.032428 -0.032428 -0.032428 -0.032428 -0.014984 0 0 0 0
  spline S89 degree 3 poles (-17.5046, 0.9246) (-17.4728, 0.8875) (-17.4061, 0.8098) (-17.3991, 0.7074) (-17.3954, 0.6538) knots -0.029902 -0.029902 -0.029902 -0.029902 -0.015625 0 0 0 0
  spline S90 degree 3 poles (-17.3954, 0.6538) (-17.3967, 0.6215) (-17.3993, 0.5593) (-17.4226, 0.5016) (-17.4338, 0.4738) knots -0.018528 -0.018528 -0.018528 -0.018528 -0.008903 0 0 0 0
  spline S91 degree 3 poles (-17.4338, 0.4738) (-17.449, 0.4484) (-17.4804, 0.3955) (-17.5298, 0.3589) (-17.5554, 0.34) knots -0.018242 -0.018242 -0.018242 -0.018242 -0.009441 0 0 0 0
  spline S92 degree 3 poles (-17.5554, 0.34) (-17.5866, 0.3224) (-17.6543, 0.2843) (-17.73, 0.2665) (-17.7708, 0.2569) knots -0.023188 -0.023188 -0.023188 -0.023188 -0.012489 0 0 0 0
  spline S93 degree 3 poles (-17.7708, 0.2569) (-17.8194, 0.2489) (-17.9253, 0.2313) (-18.0327, 0.23) (-18.0908, 0.2292) knots -0.032161 -0.032161 -0.032161 -0.032161 -0.017398 0 0 0 0
  line L18 (-18.0908, 0.2292) -> (-18.3862, 0.2292)
  line L19 (-16.0354, 1.3954) -> (-16.0354, -2.6508)
  spline S94 degree 3 poles (-16.0354, -2.6508) (-16.0346, -2.6608) (-16.0331, -2.6808) (-16.0223, -2.6977) (-16.0169, -2.7062) knots -0.005919 -0.005919 -0.005919 -0.005919 -0.002959 0 0 0 0
  spline S95 degree 3 poles (-16.0169, -2.7062) (-16.009, -2.7143) (-15.991, -2.7327) (-15.9672, -2.7423) (-15.9538, -2.7477) knots -0.007625 -0.007625 -0.007625 -0.007625 -0.004249 0 0 0 0
  spline S96 degree 3 poles (-15.9538, -2.7477) (-15.9366, -2.7531) (-15.898, -2.7654) (-15.8577, -2.7708) (-15.8354, -2.7738) knots -0.012151 -0.012151 -0.012151 -0.012151 -0.006747 0 0 0 0
  spline S97 degree 3 poles (-15.8354, -2.7738) (-15.8075, -2.7765) (-15.745, -2.7825) (-15.6823, -2.7829) (-15.6477, -2.7831) knots -0.0188 -0.0188 -0.0188 -0.0188 -0.010387 0 0 0 0
  spline S98 degree 3 poles (-15.6477, -2.7831) (-15.613, -2.7829) (-15.5503, -2.7825) (-15.4879, -2.7765) (-15.46, -2.7738) knots -0.0188 -0.0188 -0.0188 -0.0188 -0.008413 0 0 0 0
  spline S99 degree 3 poles (-15.46, -2.7738) (-15.4377, -2.7708) (-15.3974, -2.7654) (-15.3587, -2.7531) (-15.3415, -2.7477) knots -0.012151 -0.012151 -0.012151 -0.012151 -0.005405 0 0 0 0
  spline S100 degree 3 poles (-15.3415, -2.7477) (-15.3282, -2.7423) (-15.3043, -2.7327) (-15.2864, -2.7143) (-15.2785, -2.7062) knots -0.007625 -0.007625 -0.007625 -0.007625 -0.003376 0 0 0 0
  spline S101 degree 3 poles (-15.2785, -2.7062) (-15.2731, -2.6977) (-15.2623, -2.6808) (-15.2608, -2.6608) (-15.26, -2.6508) knots -0.005919 -0.005919 -0.005919 -0.005919 -0.002959 0 0 0 0
  line L20 (-15.26, -2.6508) -> (-15.26, 1.3954)
  spline S102 degree 3 poles (-15.26, 1.3954) (-15.2607, 1.4053) (-15.2622, 1.4248) (-15.2731, 1.4412) (-15.2785, 1.4492) knots -0.005779 -0.005779 -0.005779 -0.005779 -0.002858 0 0 0 0
  spline S103 degree 3 poles (-15.2785, 1.4492) (-15.2864, 1.4568) (-15.3046, 1.4742) (-15.3283, 1.4828) (-15.3415, 1.4877) knots -0.007458 -0.007458 -0.007458 -0.007458 -0.004183 0 0 0 0
  spline S104 degree 3 poles (-15.3415, 1.4877) (-15.3588, 1.4926) (-15.3976, 1.5037) (-15.4377, 1.5082) (-15.46, 1.5108) knots -0.012087 -0.012087 -0.012087 -0.012087 -0.006723 0 0 0 0
  spline S105 degree 3 poles (-15.46, 1.5108) (-15.4879, 1.513) (-15.5504, 1.518) (-15.6131, 1.5183) (-15.6477, 1.5185) knots -0.018791 -0.018791 -0.018791 -0.018791 -0.010386 0 0 0 0
  spline S106 degree 3 poles (-15.6477, 1.5185) (-15.6823, 1.5183) (-15.745, 1.518) (-15.8074, 1.513) (-15.8354, 1.5108) knots -0.018791 -0.018791 -0.018791 -0.018791 -0.008404 0 0 0 0
  spline S107 degree 3 poles (-15.8354, 1.5108) (-15.8577, 1.5082) (-15.8978, 1.5037) (-15.9366, 1.4926) (-15.9538, 1.4877) knots -0.012087 -0.012087 -0.012087 -0.012087 -0.005364 0 0 0 0
  spline S108 degree 3 poles (-15.9538, 1.4877) (-15.9671, 1.4828) (-15.9908, 1.4742) (-16.0089, 1.4568) (-16.0169, 1.4492) knots -0.007458 -0.007458 -0.007458 -0.007458 -0.003275 0 0 0 0
  spline S109 degree 3 poles (-16.0169, 1.4492) (-16.0223, 1.4412) (-16.0332, 1.4248) (-16.0346, 1.4053) (-16.0354, 1.3954) knots -0.005779 -0.005779 -0.005779 -0.005779 -0.002921 0 0 0 0
  line L21 (-25.9215, 1.3954) -> (-25.9215, -0.2877)
  spline S110 degree 3 poles (-25.9215, -0.2877) (-25.9202, -0.382) (-25.9176, -0.5564) (-25.8845, -0.7275) (-25.8692, -0.8062) knots -0.0522 -0.0522 -0.0522 -0.0522 -0.023977 0 0 0 0
  spline S111 degree 3 poles (-25.8692, -0.8062) (-25.8496, -0.8745) (-25.8112, -1.0076) (-25.7354, -1.1235) (-25.6985, -1.18) knots -0.041307 -0.041307 -0.041307 -0.041307 -0.020119 0 0 0 0
  spline S112 degree 3 poles (-25.6985, -1.18) (-25.6553, -1.2308) (-25.5675, -1.3342) (-25.4483, -1.3992) (-25.3877, -1.4323) knots -0.040335 -0.040335 -0.040335 -0.040335 -0.020531 0 0 0 0
  spline S113 degree 3 poles (-25.3877, -1.4323) (-25.3171, -1.4592) (-25.1651, -1.517) (-25.0024, -1.522) (-24.9154, -1.5246) knots -0.048425 -0.048425 -0.048425 -0.048425 -0.025911 0 0 0 0
  spline S114 degree 3 poles (-24.9154, -1.5246) (-24.841, -1.5205) (-24.6916, -1.5122) (-24.5528, -1.456) (-24.4831, -1.4277) knots -0.044576 -0.044576 -0.044576 -0.044576 -0.022404 0 0 0 0
  spline S115 degree 3 poles (-24.4831, -1.4277) (-24.4126, -1.3897) (-24.264, -1.3095) (-24.1404, -1.1944) (-24.0754, -1.1338) knots -0.050438 -0.050438 -0.050438 -0.050438 -0.02652 0 0 0 0
  line L22 (-24.0754, -1.1338) -> (-24.0754, -2.6508)
  spline S116 degree 3 poles (-24.0754, -2.6508) (-24.0746, -2.6608) (-24.0731, -2.6808) (-24.0623, -2.6977) (-24.0569, -2.7062) knots -0.005919 -0.005919 -0.005919 -0.005919 -0.002959 0 0 0 0
  spline S117 degree 3 poles (-24.0569, -2.7062) (-24.049, -2.7143) (-24.031, -2.7327) (-24.0072, -2.7423) (-23.9938, -2.7477) knots -0.007625 -0.007625 -0.007625 -0.007625 -0.004249 0 0 0 0
  spline S118 degree 3 poles (-23.9938, -2.7477) (-23.9766, -2.7531) (-23.938, -2.7654) (-23.8977, -2.7708) (-23.8754, -2.7738) knots -0.012151 -0.012151 -0.012151 -0.012151 -0.006747 0 0 0 0
  spline S119 degree 3 poles (-23.8754, -2.7738) (-23.8475, -2.7765) (-23.785, -2.7825) (-23.7223, -2.7829) (-23.6877, -2.7831) knots -0.0188 -0.0188 -0.0188 -0.0188 -0.010387 0 0 0 0
  spline S120 degree 3 poles (-23.6877, -2.7831) (-23.653, -2.7829) (-23.5903, -2.7825) (-23.5279, -2.7765) (-23.5, -2.7738) knots -0.0188 -0.0188 -0.0188 -0.0188 -0.008413 0 0 0 0
  spline S121 degree 3 poles (-23.5, -2.7738) (-23.4777, -2.7708) (-23.4374, -2.7654) (-23.3987, -2.7531) (-23.3815, -2.7477) knots -0.012151 -0.012151 -0.012151 -0.012151 -0.005405 0 0 0 0
  spline S122 degree 3 poles (-23.3815, -2.7477) (-23.3682, -2.7423) (-23.3443, -2.7327) (-23.3264, -2.7143) (-23.3185, -2.7062) knots -0.007625 -0.007625 -0.007625 -0.007625 -0.003376 0 0 0 0
  spline S123 degree 3 poles (-23.3185, -2.7062) (-23.3131, -2.6977) (-23.3023, -2.6808) (-23.3008, -2.6608) (-23.3, -2.6508) knots -0.005919 -0.005919 -0.005919 -0.005919 -0.002959 0 0 0 0
  line L23 (-23.3, -2.6508) -> (-23.3, 1.3954)
  spline S124 degree 3 poles (-23.3, 1.3954) (-23.3007, 1.4053) (-23.3022, 1.4248) (-23.3131, 1.4412) (-23.3185, 1.4492) knots -0.005779 -0.005779 -0.005779 -0.005779 -0.002858 0 0 0 0
  spline S125 degree 3 poles (-23.3185, 1.4492) (-23.3264, 1.4568) (-23.3446, 1.4742) (-23.3683, 1.4828) (-23.3815, 1.4877) knots -0.007457 -0.007457 -0.007457 -0.007457 -0.004182 0 0 0 0
  spline S126 degree 3 poles (-23.3815, 1.4877) (-23.3988, 1.4926) (-23.4376, 1.5037) (-23.4777, 1.5082) (-23.5, 1.5108) knots -0.012087 -0.012087 -0.012087 -0.012087 -0.006723 0 0 0 0
  spline S127 degree 3 poles (-23.5, 1.5108) (-23.5279, 1.513) (-23.5904, 1.518) (-23.6531, 1.5183) (-23.6877, 1.5185) knots -0.018791 -0.018791 -0.018791 -0.018791 -0.010387 0 0 0 0
  spline S128 degree 3 poles (-23.6877, 1.5185) (-23.7223, 1.5183) (-23.785, 1.518) (-23.8475, 1.513) (-23.8754, 1.5108) knots -0.018791 -0.018791 -0.018791 -0.018791 -0.008405 0 0 0 0
  spline S129 degree 3 poles (-23.8754, 1.5108) (-23.8977, 1.5082) (-23.9378, 1.5037) (-23.9766, 1.4926) (-23.9938, 1.4877) knots -0.012087 -0.012087 -0.012087 -0.012087 -0.005364 0 0 0 0
  spline S130 degree 3 poles (-23.9938, 1.4877) (-24.0071, 1.4828) (-24.0308, 1.4742) (-24.0489, 1.4568) (-24.0569, 1.4492) knots -0.007457 -0.007457 -0.007457 -0.007457 -0.003275 0 0 0 0
  spline S131 degree 3 poles (-24.0569, 1.4492) (-24.0623, 1.4412) (-24.0732, 1.4248) (-24.0747, 1.4053) (-24.0754, 1.3954) knots -0.005779 -0.005779 -0.005779 -0.005779 -0.002921 0 0 0 0
  line L24 (-24.0754, 1.3954) -> (-24.0754, -0.4292)
  spline S132 degree 3 poles (-24.0754, -0.4292) (-24.1266, -0.4919) (-24.2207, -0.6071) (-24.3365, -0.7005) (-24.3892, -0.7431) knots -0.04449 -0.04449 -0.04449 -0.04449 -0.020291 0 0 0 0
  spline S133 degree 3 poles (-24.3892, -0.7431) (-24.4377, -0.7745) (-24.529, -0.8336) (-24.637, -0.8453) (-24.6877, -0.8508) knots -0.032125 -0.032125 -0.032125 -0.032125 -0.015088 0 0 0 0
  spline S134 degree 3 poles (-24.6877, -0.8508) (-24.7247, -0.8493) (-24.7956, -0.8464) (-24.8611, -0.8192) (-24.8923, -0.8062) knots -0.02109 -0.02109 -0.02109 -0.02109 -0.010072 0 0 0 0
  spline S135 degree 3 poles (-24.8923, -0.8062) (-24.9202, -0.7897) (-24.976, -0.7569) (-25.0156, -0.7056) (-25.0354, -0.68) knots -0.019232 -0.019232 -0.019232 -0.019232 -0.009621 0 0 0 0
  spline S136 degree 3 poles (-25.0354, -0.68) (-25.053, -0.6507) (-25.0897, -0.5893) (-25.1096, -0.5205) (-25.12, -0.4846) knots -0.021372 -0.021372 -0.021372 -0.021372 -0.011165 0 0 0 0
  spline S137 degree 3 poles (-25.12, -0.4846) (-25.1285, -0.4396) (-25.148, -0.336) (-25.1488, -0.2305) (-25.1492, -0.1708) knots -0.031576 -0.031576 -0.031576 -0.031576 -0.017861 0 0 0 0
  line L25 (-25.1492, -0.1708) -> (-25.1492, 1.3954)
  spline S138 degree 3 poles (-25.1492, 1.3954) (-25.15, 1.4053) (-25.1514, 1.4248) (-25.1623, 1.4412) (-25.1677, 1.4492) knots -0.005779 -0.005779 -0.005779 -0.005779 -0.002858 0 0 0 0
  spline S139 degree 3 poles (-25.1677, 1.4492) (-25.1755, 1.4568) (-25.1933, 1.474) (-25.2164, 1.4828) (-25.2292, 1.4877) knots -0.007323 -0.007323 -0.007323 -0.007323 -0.004078 0 0 0 0
  spline S140 degree 3 poles (-25.2292, 1.4877) (-25.2462, 1.4926) (-25.285, 1.5039) (-25.3251, 1.5083) (-25.3477, 1.5108) knots -0.012089 -0.012089 -0.012089 -0.012089 -0.006799 0 0 0 0
  spline S141 degree 3 poles (-25.3477, 1.5108) (-25.376, 1.513) (-25.439, 1.518) (-25.5022, 1.5183) (-25.5369, 1.5185) knots -0.018944 -0.018944 -0.018944 -0.018944 -0.010425 0 0 0 0
  spline S142 degree 3 poles (-25.5369, 1.5185) (-25.5709, 1.5183) (-25.6331, 1.5179) (-25.695, 1.513) (-25.7231, 1.5108) knots -0.018637 -0.018637 -0.018637 -0.018637 -0.008443 0 0 0 0
  spline S143 degree 3 poles (-25.7231, 1.5108) (-25.7457, 1.5083) (-25.7858, 1.5039) (-25.8246, 1.4926) (-25.8415, 1.4877) knots -0.012089 -0.012089 -0.012089 -0.012089 -0.005289 0 0 0 0
  spline S144 degree 3 poles (-25.8415, 1.4877) (-25.8544, 1.4828) (-25.8775, 1.474) (-25.8952, 1.4568) (-25.9031, 1.4492) knots -0.007323 -0.007323 -0.007323 -0.007323 -0.003246 0 0 0 0
  spline S145 degree 3 poles (-25.9031, 1.4492) (-25.9085, 1.4412) (-25.9193, 1.4248) (-25.9208, 1.4053) (-25.9215, 1.3954) knots -0.005779 -0.005779 -0.005779 -0.005779 -0.002921 0 0 0 0
  point P0 (-22.95, -6.1)
  point P1 (-23.35, -5.1)
  point P2 (-29.15, -5.6164)
  point P3 (-23.95, -6.1)
  point P4 (-24.35, -5.1)
  dimension "d48" = 0.5
  dimension "d49" = 0.5
  dimension "d50" = 0.448
  dimension "d51" = 0.448
  dimension "d52" = 0.4
  dimension "d56" = -1
  dimension "d57" = 0
  constraint coincident P4 L4.start
  constraint coincident P0 L2.end
  constraint coincident P1 L5.start
  constraint coincident P3 L3.end
  constraint equal L2 L4
  constraint equal L3 L5
  constraint equal L0 L6
  constraint perpendicular L1 L6
  constraint parallel L0 L6
  measures "d48" distance of L1 P0
  measures "d49" distance of L1 P1
  measures "d50" distance of S0.start P0
  measures "d51" distance of P1 S0.end
  measures "d52" horizontal distance of P0 P1
extrude "Extrusion5" [suppressed]
move_body "Verschieben1" [suppressed]
combine "Kombinieren1" [suppressed]
equation "d525 = 0.0 °"
equation "d4 = ( 37.8 / 2 ) * 1 mm + ( ( Box_width - 1 ) * 42 / 2 ) * 1 mm"
equation "M = 2" comment "Nominal thread diameter"
equation "Box_width = 2"
equation "d26 = head_diameter_dk / 2"
equation "bolt_length_l = 6 mm" comment "bolt length"
equation "head_length_k = 3 mm"
equation "head_diameter_dk = 5 mm"
equation "total_bolt_length = drawn_bolt_length + head_length_k"
equation "Hex_width = 3 mm"
equation "distance_bolt_head_to_head_view = 1.5 mm"
equation "total_pic_width = total_bolt_length + head_diameter_dk + distance_bolt_head_to_head_view"
equation "head_corner_R = 0.3 mm"
equation "P = 0.5 mm" comment "Pitch"
equation "d64 = if(Broken_bolt == 1; broken_bolt_length / 2; 0 mm)"
equation "Broken_bolt = if(drawn_bolt_length == bolt_length_l; 0; 1)" comment "1 to split bolt pic, 0 to keep it"
equation "drawn_bolt_length = ( if(head_diameter_dk + distance_bolt_head_to_head_view + head_length_k + bolt_length_l > d4 * 2 - 5 mm; broken_bolt_length; bolt_length_l) )"
equation "M_drawn = 2.5 mm"
equation "label_text = 0" comment "M2"
equation "part_vews_distance = head_diameter_dk / 2 + distance_bolt_head_to_head_view" comment "distance between top and side views of part"
equation "broken_bolt_length = d4 * 2 - 10 mm - head_diameter_dk - distance_bolt_head_to_head_view"
